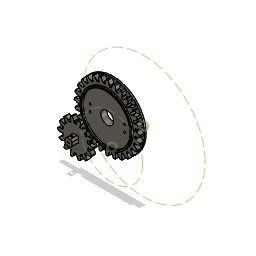
Gears v2 v7 (Autodesk Fusion 360 design; units mm, degrees)
description: Spur Gear; Module: 12.7; Num Teeth: 28; Pressure Angle: 20.0; Backlash: 0.00 mm
description: Spur Gear; Module: 12.7; Num Teeth: 14; Pressure Angle: 20.0; Backlash: 0.00 mm
Autodesk Fusion 360 part; units mm, degrees
(part 1 of 11)
sketch "Sketch1" plane through (0, 0, 0) normal (0, 0, 1) x (1, 0, 0)
  line L0 (-152.4, 152.4) -> (152.4, 152.4)
  line L1 (152.4, 152.4) -> (152.4, -152.4)
  line L2 (152.4, -152.4) -> (-152.4, -152.4)
  line L3 (-152.4, -152.4) -> (-152.4, 152.4)
  line L4 (-152.4, 152.4) -> (152.4, -152.4)
  dimension "d25" = 304.8
  dimension "d26" = 304.8
  constraint horizontal L0
  constraint vertical L1
  constraint horizontal L2
  constraint vertical L3
  constraint midpoint origin L4
  measures "d25" distance of L0.start L0.end
  measures "d26" distance of L0.end L1.end
sketch "Sketch1 (2)" plane through (0, 0, 0) normal (0, 0, 1) x (1, 0, 0) in component "Spur Gear (28 teeth)"
  circle A0 centre (0, 0) radius 162.5092
  circle A1 centre (0, 0) radius 31
extrude "Extrude1" add sketch "Sketch1 (2)" along normal blind 25 makes body 1 in component "Spur Gear (28 teeth)"
sketch "Sketch2" plane through (0, 0, 0) normal (0, 0, 1) x (1, 0, 0) in component "Spur Gear (28 teeth)"
  spline S0 degree 5 poles (166.6564, -11.8532) (166.7254, -11.8581) (166.8636, -11.8663) (167.071, -11.8735) (167.3475, -11.8735) (167.6934, -11.8606) (168.0395, -11.8383) (168.3856, -11.8103) (168.7317, -11.7791) (169.0778, -11.7459) (169.4239, -11.7106) (169.7699, -11.6722) (170.1158, -11.63) (170.4617, -11.5833) (170.8074, -11.5321) (171.153, -11.4767) (171.4984, -11.4177) (171.8437, -11.3558) (172.1889, -11.2914) (172.5338, -11.2245) (172.8787, -11.1552) (173.2233, -11.0833) (173.5677, -11.0087) (173.912, -10.9313) (174.256, -10.8512) (174.5999, -10.7684) (174.9435, -10.6832) (175.2869, -10.5956) (175.6301, -10.5057) (175.973, -10.4136) (176.3158, -10.3193) (176.6582, -10.2229) (177.0005, -10.1242) (177.3424, -10.0233) (177.6842, -9.9203) (178.0256, -9.8151) (178.3669, -9.7079) (178.7078, -9.5986) (179.0485, -9.4873) (179.3888, -9.374) (179.729, -9.2588) (180.0688, -9.1417) (180.4083, -9.0226) (180.7476, -8.9017) (181.0865, -8.7788) (181.4252, -8.6541) (181.7635, -8.5275) (182.1016, -8.3991) (182.4393, -8.269) (182.7767, -8.137) (183.1138, -8.0033) (183.4506, -7.8678) (183.7871, -7.7306) (184.1232, -7.5916) (184.459, -7.451) (184.7945, -7.3086) (185.1296, -7.1646) (185.4644, -7.0189) (185.7989, -6.8716) (186.133, -6.7226) (186.4667, -6.572) (186.8001, -6.4197) (187.1332, -6.2659) (187.4659, -6.1105) (187.7982, -5.9535) (188.1302, -5.7949) (188.4618, -5.6348) (188.793, -5.4731) (189.1239, -5.3099) (189.4544, -5.1452) (189.7845, -4.979) (190.0482, -4.8448) (190.2459, -4.7434) (190.3776, -4.6756) (190.4434, -4.6415) knots 0 0 0 0 0 0 0.01428571 0.02857143 0.04285714 0.05714286 0.07142857 0.08571429 0.1 0.11428571 0.12857143 0.14285714 0.15714286 0.17142857 0.18571429 0.2 0.21428571 0.22857143 0.24285714 0.25714286 0.27142857 0.28571429 0.3 0.31428571 0.32857143 0.34285714 0.35714286 0.37142857 0.38571429 0.4 0.41428571 0.42857143 0.44285714 0.45714286 0.47142857 0.48571429 0.5 0.51428571 0.52857143 0.54285714 0.55714286 0.57142857 0.58571429 0.6 0.61428571 0.62857143 0.64285714 0.65714286 0.67142857 0.68571429 0.7 0.71428571 0.72857143 0.74285714 0.75714286 0.77142857 0.78571429 0.8 0.81428571 0.82857143 0.84285714 0.85714286 0.87142857 0.88571429 0.9 0.91428571 0.92857143 0.94285714 0.95714286 0.97142857 0.98571429 1 1 1 1 1 1
  spline S1 degree 5 poles (166.6564, 11.8532) (166.7254, 11.8581) (166.8636, 11.8663) (167.071, 11.8735) (167.3475, 11.8735) (167.6934, 11.8606) (168.0395, 11.8383) (168.3856, 11.8103) (168.7317, 11.7791) (169.0778, 11.7459) (169.4239, 11.7106) (169.7699, 11.6722) (170.1158, 11.63) (170.4617, 11.5833) (170.8074, 11.5321) (171.153, 11.4767) (171.4984, 11.4177) (171.8437, 11.3558) (172.1889, 11.2914) (172.5338, 11.2245) (172.8787, 11.1552) (173.2233, 11.0833) (173.5677, 11.0087) (173.912, 10.9313) (174.256, 10.8512) (174.5999, 10.7684) (174.9435, 10.6832) (175.2869, 10.5956) (175.6301, 10.5057) (175.973, 10.4136) (176.3158, 10.3193) (176.6582, 10.2229) (177.0005, 10.1242) (177.3424, 10.0233) (177.6842, 9.9203) (178.0256, 9.8151) (178.3669, 9.7079) (178.7078, 9.5986) (179.0485, 9.4873) (179.3888, 9.374) (179.729, 9.2588) (180.0688, 9.1417) (180.4083, 9.0226) (180.7476, 8.9017) (181.0865, 8.7788) (181.4252, 8.6541) (181.7635, 8.5275) (182.1016, 8.3991) (182.4393, 8.269) (182.7767, 8.137) (183.1138, 8.0033) (183.4506, 7.8678) (183.7871, 7.7306) (184.1232, 7.5916) (184.459, 7.451) (184.7945, 7.3086) (185.1296, 7.1646) (185.4644, 7.0189) (185.7989, 6.8716) (186.133, 6.7226) (186.4667, 6.572) (186.8001, 6.4197) (187.1332, 6.2659) (187.4659, 6.1105) (187.7982, 5.9535) (188.1302, 5.7949) (188.4618, 5.6348) (188.793, 5.4731) (189.1239, 5.3099) (189.4544, 5.1452) (189.7845, 4.979) (190.0482, 4.8448) (190.2459, 4.7434) (190.3776, 4.6756) (190.4434, 4.6415) knots 0 0 0 0 0 0 0.01428571 0.02857143 0.04285714 0.05714286 0.07142857 0.08571429 0.1 0.11428571 0.12857143 0.14285714 0.15714286 0.17142857 0.18571429 0.2 0.21428571 0.22857143 0.24285714 0.25714286 0.27142857 0.28571429 0.3 0.31428571 0.32857143 0.34285714 0.35714286 0.37142857 0.38571429 0.4 0.41428571 0.42857143 0.44285714 0.45714286 0.47142857 0.48571429 0.5 0.51428571 0.52857143 0.54285714 0.55714286 0.57142857 0.58571429 0.6 0.61428571 0.62857143 0.64285714 0.65714286 0.67142857 0.68571429 0.7 0.71428571 0.72857143 0.74285714 0.75714286 0.77142857 0.78571429 0.8 0.81428571 0.82857143 0.84285714 0.85714286 0.87142857 0.88571429 0.9 0.91428571 0.92857143 0.94285714 0.95714286 0.97142857 0.98571429 1 1 1 1 1 1
  arc A0 (190.4434, -4.6415) -> (190.4434, 4.6415) centre (0, 0) ccw
  line L0 (162.0897, -11.5292) -> (166.6564, -11.8532)
  line L1 (162.0897, 11.5292) -> (166.6564, 11.8532)
  line L2 (162.0897, -11.5292) -> (162.0897, 11.5292)
  point P0 (168.3364, -11.8136)
  point P1 (170.0254, -11.6404)
  point P2 (171.72, -11.3777)
  point P3 (173.4184, -11.0406)
  point P4 (175.1198, -10.6379)
  point P5 (176.8231, -10.175)
  point P6 (178.5277, -9.656)
  point P7 (180.2329, -9.0839)
  point P8 (181.9381, -8.461)
  point P9 (183.6427, -7.7892)
  point P10 (185.3461, -7.0702)
  point P11 (187.0477, -6.3051)
  point P12 (188.747, -5.4953)
  point P13 (168.3364, 11.8136)
  point P14 (170.0254, 11.6404)
  point P15 (171.72, 11.3777)
  point P16 (173.4184, 11.0406)
  point P17 (175.1198, 10.6379)
  point P18 (176.8231, 10.175)
  point P19 (178.5277, 9.656)
  point P20 (180.2329, 9.0839)
  point P21 (181.9381, 8.461)
  point P22 (183.6427, 7.7892)
  point P23 (185.3461, 7.0702)
  point P24 (187.0477, 6.3051)
  point P25 (188.747, 5.4953)
extrude "Extrude2" add sketch "Sketch2" along normal blind 25 bodies 1 in component "Spur Gear (28 teeth)"
fillet "Fillet1" radius 1.5875 2 edges at (162.0997, -11.5299, 12.5) (162.0997, 11.5299, 12.5) on bodies 1 in component "Spur Gear (28 teeth)"
pattern_circular "C-Pattern1" count 28 over 360 about axis through (0, 0, 0) along (0, 0, 1) of "Extrude2", "Fillet1" in component "Spur Gear (28 teeth)"
sketch "Sketch3" plane through (0, 0, 0) normal (0, 0, 1) x (1, 0, 0) in component "Spur Gear (28 teeth)"
  circle A0 centre (0, 0) radius 177.8 construction
sketch "Sketch1 (3)" plane through (0, 0, 0) normal (0, 0, 1) x (1, 0, 0) in component "Spur Gear (14 teeth)"
  circle A0 centre (0, 0) radius 73.6092
  circle A1 centre (0, 0) radius 10
extrude "Extrude1'" add sketch "Sketch1 (3)" along normal blind 25 separate body makes body 2 in component "Spur Gear (14 teeth)"
sketch "Sketch2 (2)" plane through (0, 0, 0) normal (0, 0, 1) x (1, 0, 0) in component "Spur Gear (14 teeth)"
  spline S0 degree 5 poles (82.8648, -10.5895) (82.9186, -10.5964) (83.0264, -10.6085) (83.1884, -10.6217) (83.4049, -10.6299) (83.6763, -10.6275) (83.9482, -10.6159) (84.2204, -10.5989) (84.4927, -10.5788) (84.7651, -10.5568) (85.0375, -10.5325) (85.31, -10.5051) (85.5825, -10.4738) (85.855, -10.438) (86.1276, -10.3977) (86.4002, -10.3533) (86.6727, -10.3055) (86.9452, -10.2547) (87.2175, -10.2014) (87.4897, -10.1457) (87.7618, -10.0875) (88.0338, -10.0267) (88.3056, -9.9631) (88.5772, -9.8967) (88.8487, -9.8275) (89.12, -9.7558) (89.3911, -9.6815) (89.6621, -9.6048) (89.9328, -9.5259) (90.2032, -9.4447) (90.4735, -9.3613) (90.7435, -9.2757) (91.0132, -9.1878) (91.2827, -9.0976) (91.5519, -9.0053) (91.8209, -8.9108) (92.0895, -8.8142) (92.3579, -8.7155) (92.626, -8.6148) (92.8938, -8.5121) (93.1612, -8.4074) (93.4284, -8.3007) (93.6952, -8.192) (93.9617, -8.0814) (94.2278, -7.9688) (94.4936, -7.8544) (94.7591, -7.738) (95.0241, -7.6198) (95.2889, -7.4998) (95.5532, -7.3779) (95.8172, -7.2542) (96.0808, -7.1287) (96.3439, -7.0014) (96.6067, -6.8723) (96.8691, -6.7415) (97.1311, -6.6089) (97.3927, -6.4747) (97.6539, -6.3387) (97.9146, -6.201) (98.1749, -6.0616) (98.4348, -5.9205) (98.6942, -5.7778) (98.9532, -5.6334) (99.2117, -5.4874) (99.4698, -5.3397) (99.7274, -5.1905) (99.9845, -5.0396) (100.2412, -4.8871) (100.4974, -4.7331) (100.7531, -4.5775) (101.0083, -4.4203) (101.2121, -4.2933) (101.3647, -4.1974) (101.4664, -4.1331) (101.5172, -4.1009) knots 0 0 0 0 0 0 0.01428571 0.02857143 0.04285714 0.05714286 0.07142857 0.08571429 0.1 0.11428571 0.12857143 0.14285714 0.15714286 0.17142857 0.18571429 0.2 0.21428571 0.22857143 0.24285714 0.25714286 0.27142857 0.28571429 0.3 0.31428571 0.32857143 0.34285714 0.35714286 0.37142857 0.38571429 0.4 0.41428571 0.42857143 0.44285714 0.45714286 0.47142857 0.48571429 0.5 0.51428571 0.52857143 0.54285714 0.55714286 0.57142857 0.58571429 0.6 0.61428571 0.62857143 0.64285714 0.65714286 0.67142857 0.68571429 0.7 0.71428571 0.72857143 0.74285714 0.75714286 0.77142857 0.78571429 0.8 0.81428571 0.82857143 0.84285714 0.85714286 0.87142857 0.88571429 0.9 0.91428571 0.92857143 0.94285714 0.95714286 0.97142857 0.98571429 1 1 1 1 1 1
  spline S1 degree 5 poles (82.8648, 10.5895) (82.9186, 10.5964) (83.0264, 10.6085) (83.1884, 10.6217) (83.4049, 10.6299) (83.6763, 10.6275) (83.9482, 10.6159) (84.2204, 10.5989) (84.4927, 10.5788) (84.7651, 10.5568) (85.0375, 10.5325) (85.31, 10.5051) (85.5825, 10.4738) (85.855, 10.438) (86.1276, 10.3977) (86.4002, 10.3533) (86.6727, 10.3055) (86.9452, 10.2547) (87.2175, 10.2014) (87.4897, 10.1457) (87.7618, 10.0875) (88.0338, 10.0267) (88.3056, 9.9631) (88.5772, 9.8967) (88.8487, 9.8275) (89.12, 9.7558) (89.3911, 9.6815) (89.6621, 9.6048) (89.9328, 9.5259) (90.2032, 9.4447) (90.4735, 9.3613) (90.7435, 9.2757) (91.0132, 9.1878) (91.2827, 9.0976) (91.5519, 9.0053) (91.8209, 8.9108) (92.0895, 8.8142) (92.3579, 8.7155) (92.626, 8.6148) (92.8938, 8.5121) (93.1612, 8.4074) (93.4284, 8.3007) (93.6952, 8.192) (93.9617, 8.0814) (94.2278, 7.9688) (94.4936, 7.8544) (94.7591, 7.738) (95.0241, 7.6198) (95.2889, 7.4998) (95.5532, 7.3779) (95.8172, 7.2542) (96.0808, 7.1287) (96.3439, 7.0014) (96.6067, 6.8723) (96.8691, 6.7415) (97.1311, 6.6089) (97.3927, 6.4747) (97.6539, 6.3387) (97.9146, 6.201) (98.1749, 6.0616) (98.4348, 5.9205) (98.6942, 5.7778) (98.9532, 5.6334) (99.2117, 5.4874) (99.4698, 5.3397) (99.7274, 5.1905) (99.9845, 5.0396) (100.2412, 4.8871) (100.4974, 4.7331) (100.7531, 4.5775) (101.0083, 4.4203) (101.2121, 4.2933) (101.3647, 4.1974) (101.4664, 4.1331) (101.5172, 4.1009) knots 0 0 0 0 0 0 0.01428571 0.02857143 0.04285714 0.05714286 0.07142857 0.08571429 0.1 0.11428571 0.12857143 0.14285714 0.15714286 0.17142857 0.18571429 0.2 0.21428571 0.22857143 0.24285714 0.25714286 0.27142857 0.28571429 0.3 0.31428571 0.32857143 0.34285714 0.35714286 0.37142857 0.38571429 0.4 0.41428571 0.42857143 0.44285714 0.45714286 0.47142857 0.48571429 0.5 0.51428571 0.52857143 0.54285714 0.55714286 0.57142857 0.58571429 0.6 0.61428571 0.62857143 0.64285714 0.65714286 0.67142857 0.68571429 0.7 0.71428571 0.72857143 0.74285714 0.75714286 0.77142857 0.78571429 0.8 0.81428571 0.82857143 0.84285714 0.85714286 0.87142857 0.88571429 0.9 0.91428571 0.92857143 0.94285714 0.95714286 0.97142857 0.98571429 1 1 1 1 1 1
  arc A0 (101.5172, -4.1009) -> (101.5172, 4.1009) centre (0, 0) ccw
  line L0 (73.0055, -9.3309) -> (82.8648, -10.5895)
  line L1 (73.0055, 9.3309) -> (82.8648, 10.5895)
  line L2 (73.0055, -9.3309) -> (73.0055, 9.3309)
  point P0 (84.1637, -10.6019)
  point P1 (85.4782, -10.4853)
  point P2 (86.8022, -10.281)
  point P3 (88.1332, -10.003)
  point P4 (89.4693, -9.659)
  point P5 (90.8089, -9.254)
  point P6 (92.1509, -8.7913)
  point P7 (93.4941, -8.2736)
  point P8 (94.8372, -7.7029)
  point P9 (96.1793, -7.0807)
  point P10 (97.5194, -6.4084)
  point P11 (98.8564, -5.6871)
  point P12 (100.1893, -4.9177)
  point P13 (84.1637, 10.6019)
  point P14 (85.4782, 10.4853)
  point P15 (86.8022, 10.281)
  point P16 (88.1332, 10.003)
  point P17 (89.4693, 9.659)
  point P18 (90.8089, 9.254)
  point P19 (92.1509, 8.7913)
  point P20 (93.4941, 8.2736)
  point P21 (94.8372, 7.7029)
  point P22 (96.1793, 7.0807)
  point P23 (97.5194, 6.4084)
  point P24 (98.8564, 5.6871)
  point P25 (100.1893, 4.9177)
extrude "Extrude2'" add sketch "Sketch2 (2)" along normal blind 25 bodies 2 in component "Spur Gear (14 teeth)"
fillet "Fillet1'" radius 1.5875 2 edges at (73.0152, -9.3321, 12.5) (73.0152, 9.3321, 12.5) on bodies 2 in component "Spur Gear (14 teeth)"
pattern_circular "C-Pattern1'" count 14 over 360 about axis through (0, 0, 0) along (0, 0, 1) of "Extrude2'", "Fillet1'" in component "Spur Gear (14 teeth)"
sketch "Sketch3 (2)" plane through (0, 0, 0) normal (0, 0, 1) x (1, 0, 0) in component "Spur Gear (14 teeth)"
  circle A0 centre (0, 0) radius 88.9 construction
scale "Scale1" factor 0.5 about (-161.9806, -13.0972, 25) bodies 1 in component "Spur Gear (28 teeth)"
scale "Scale1'" factor 0.5 about (-161.9806, -13.0972, 25) bodies 2 in component "Spur Gear (14 teeth)"
sketch "Sketch2 (3)" plane through (0, 0, 25) normal (0, 0, 1) x (1, 0, 0)
  arc A0 (79.8631, -10.983) -> (80.4364, -5.894) centre (-0.5538, 0.6546) ccw
  arc A1 (81.2838, -5.1662) -> (80.4364, -5.894) centre (81.2276, -5.958) ccw
  line L0 (81.2838, -5.1662) -> (82.7743, -5.272)
  spline S0 degree 5 poles (82.7743, -5.272) (82.8089, -5.2744) (82.878, -5.2785) (82.9816, -5.2821) (83.1199, -5.2821) (83.2929, -5.2756) (83.4659, -5.2645) (83.6389, -5.2505) (83.812, -5.2349) (83.9851, -5.2183) (84.1581, -5.2006) (84.3311, -5.1815) (84.5041, -5.1604) (84.677, -5.137) (84.8498, -5.1114) (85.0226, -5.0837) (85.1954, -5.0542) (85.368, -5.0233) (85.5406, -4.991) (85.7131, -4.9576) (85.8855, -4.9229) (86.0578, -4.887) (86.23, -4.8497) (86.4021, -4.811) (86.5742, -4.7709) (86.7461, -4.7296) (86.9179, -4.6869) (87.0896, -4.6431) (87.2612, -4.5982) (87.4327, -4.5522) (87.604, -4.505) (87.7753, -4.4568) (87.9464, -4.4075) (88.1174, -4.357) (88.2882, -4.3055) (88.459, -4.2529) (88.6296, -4.1993) (88.8001, -4.1446) (88.9704, -4.089) (89.1406, -4.0324) (89.3106, -3.9748) (89.4806, -3.9162) (89.6503, -3.8567) (89.8199, -3.7962) (89.9894, -3.7348) (90.1588, -3.6724) (90.3279, -3.6091) (90.4969, -3.5449) (90.6658, -3.4798) (90.8345, -3.4139) (91.0031, -3.347) (91.1715, -3.2793) (91.3397, -3.2106) (91.5078, -3.1412) (91.6757, -3.0708) (91.8434, -2.9997) (92.011, -2.9277) (92.1784, -2.8548) (92.3456, -2.7811) (92.5127, -2.7067) (92.6795, -2.6313) (92.8462, -2.5552) (93.0128, -2.4783) (93.1791, -2.4006) (93.3453, -2.3221) (93.5113, -2.2428) (93.6771, -2.1628) (93.8427, -2.0819) (94.0081, -2.0003) (94.1733, -1.918) (94.3384, -1.8348) (94.4703, -1.7677) (94.5691, -1.7171) (94.635, -1.6831) (94.6679, -1.6661) knots 0 0 0 0 0 0 0.01428571 0.02857143 0.04285714 0.05714286 0.07142857 0.08571429 0.1 0.11428571 0.12857143 0.14285714 0.15714286 0.17142857 0.18571429 0.2 0.21428571 0.22857143 0.24285714 0.25714286 0.27142857 0.28571429 0.3 0.31428571 0.32857143 0.34285714 0.35714286 0.37142857 0.38571429 0.4 0.41428571 0.42857143 0.44285714 0.45714286 0.47142857 0.48571429 0.5 0.51428571 0.52857143 0.54285714 0.55714286 0.57142857 0.58571429 0.6 0.61428571 0.62857143 0.64285714 0.65714286 0.67142857 0.68571429 0.7 0.71428571 0.72857143 0.74285714 0.75714286 0.77142857 0.78571429 0.8 0.81428571 0.82857143 0.84285714 0.85714286 0.87142857 0.88571429 0.9 0.91428571 0.92857143 0.94285714 0.95714286 0.97142857 0.98571429 1 1 1 1 1 1
  arc A2 (94.6679, -1.6661) -> (94.6679, 2.9754) centre (-0.5538, 0.6546) ccw
  spline S1 degree 5 poles (94.6679, 2.9754) (94.635, 2.9924) (94.5691, 3.0263) (94.4703, 3.077) (94.3384, 3.1441) (94.1733, 3.2272) (94.0081, 3.3096) (93.8427, 3.3912) (93.6771, 3.472) (93.5113, 3.5521) (93.3453, 3.6314) (93.1791, 3.7099) (93.0128, 3.7876) (92.8462, 3.8645) (92.6795, 3.9406) (92.5127, 4.0159) (92.3456, 4.0904) (92.1784, 4.1641) (92.011, 4.2369) (91.8434, 4.3089) (91.6757, 4.3801) (91.5078, 4.4504) (91.3397, 4.5199) (91.1715, 4.5885) (91.0031, 4.6563) (90.8345, 4.7231) (90.6658, 4.7891) (90.4969, 4.8542) (90.3279, 4.9184) (90.1588, 4.9817) (89.9894, 5.044) (89.8199, 5.1055) (89.6503, 5.166) (89.4806, 5.2255) (89.3106, 5.2841) (89.1406, 5.3417) (88.9704, 5.3983) (88.8001, 5.4539) (88.6296, 5.5086) (88.459, 5.5622) (88.2882, 5.6148) (88.1174, 5.6663) (87.9464, 5.7167) (87.7753, 5.7661) (87.604, 5.8143) (87.4327, 5.8615) (87.2612, 5.9075) (87.0896, 5.9524) (86.9179, 5.9962) (86.7461, 6.0388) (86.5742, 6.0802) (86.4021, 6.1203) (86.23, 6.159) (86.0578, 6.1963) (85.8855, 6.2322) (85.7131, 6.2669) (85.5406, 6.3003) (85.368, 6.3326) (85.1954, 6.3635) (85.0226, 6.393) (84.8498, 6.4207) (84.677, 6.4463) (84.5041, 6.4697) (84.3311, 6.4908) (84.1581, 6.5099) (83.9851, 6.5276) (83.812, 6.5442) (83.6389, 6.5598) (83.4659, 6.5738) (83.2929, 6.5849) (83.1199, 6.5914) (82.9816, 6.5914) (82.878, 6.5878) (82.8089, 6.5837) (82.7743, 6.5813) knots -1 -1 -1 -1 -1 -1 -0.98571429 -0.97142857 -0.95714286 -0.94285714 -0.92857143 -0.91428571 -0.9 -0.88571429 -0.87142857 -0.85714286 -0.84285714 -0.82857143 -0.81428571 -0.8 -0.78571429 -0.77142857 -0.75714286 -0.74285714 -0.72857143 -0.71428571 -0.7 -0.68571429 -0.67142857 -0.65714286 -0.64285714 -0.62857143 -0.61428571 -0.6 -0.58571429 -0.57142857 -0.55714286 -0.54285714 -0.52857143 -0.51428571 -0.5 -0.48571429 -0.47142857 -0.45714286 -0.44285714 -0.42857143 -0.41428571 -0.4 -0.38571429 -0.37142857 -0.35714286 -0.34285714 -0.32857143 -0.31428571 -0.3 -0.28571429 -0.27142857 -0.25714286 -0.24285714 -0.22857143 -0.21428571 -0.2 -0.18571429 -0.17142857 -0.15714286 -0.14285714 -0.12857143 -0.11428571 -0.1 -0.08571429 -0.07142857 -0.05714286 -0.04285714 -0.02857143 -0.01428571 0 0 0 0 0 0
  line L1 (82.7743, 6.5813) -> (81.2838, 6.4755)
  arc A3 (80.4364, 7.2033) -> (81.2838, 6.4755) centre (81.2276, 7.2672) ccw
  arc A4 (80.4364, 7.2033) -> (79.8631, 12.2922) centre (-0.5538, 0.6546) ccw
  arc A5 (80.5272, 13.1903) -> (79.8631, 12.2922) centre (80.6486, 12.4059) ccw
  line L2 (80.5272, 13.1903) -> (82.0039, 13.4189)
  spline S2 degree 5 poles (82.0039, 13.4189) (82.0381, 13.4242) (82.1064, 13.4356) (82.2083, 13.4551) (82.3431, 13.4859) (82.5103, 13.5307) (82.6765, 13.5801) (82.8421, 13.6322) (83.0073, 13.6859) (83.1724, 13.7406) (83.3371, 13.7963) (83.5015, 13.8535) (83.6655, 13.9126) (83.8288, 13.9738) (83.9917, 14.0373) (84.154, 14.1027) (84.3158, 14.1699) (84.4772, 14.2385) (84.6383, 14.3083) (84.799, 14.3793) (84.9594, 14.4515) (85.1194, 14.5248) (85.279, 14.5995) (85.4382, 14.6756) (85.597, 14.7529) (85.7554, 14.8315) (85.9134, 14.9113) (86.0711, 14.9922) (86.2284, 15.0742) (86.3853, 15.1572) (86.5419, 15.2413) (86.6981, 15.3264) (86.8539, 15.4126) (87.0094, 15.4998) (87.1645, 15.5881) (87.3193, 15.6774) (87.4737, 15.7676) (87.6277, 15.8588) (87.7814, 15.9509) (87.9347, 16.044) (88.0877, 16.138) (88.2403, 16.2329) (88.3926, 16.3287) (88.5445, 16.4255) (88.6961, 16.5231) (88.8473, 16.6215) (88.9981, 16.7209) (89.1486, 16.8211) (89.2988, 16.9221) (89.4486, 17.024) (89.598, 17.1267) (89.7471, 17.2302) (89.8958, 17.3345) (90.0442, 17.4396) (90.1923, 17.5456) (90.34, 17.6523) (90.4873, 17.7598) (90.6343, 17.868) (90.7809, 17.9771) (90.9272, 18.0869) (91.0732, 18.1974) (91.2188, 18.3087) (91.364, 18.4208) (91.5089, 18.5335) (91.6534, 18.647) (91.7976, 18.7613) (91.9414, 18.8762) (92.0849, 18.9919) (92.228, 19.1082) (92.3708, 19.2253) (92.5132, 19.3431) (92.6269, 19.4379) (92.7119, 19.5092) (92.7686, 19.557) (92.7969, 19.5809) knots 0 0 0 0 0 0 0.01428571 0.02857143 0.04285714 0.05714286 0.07142857 0.08571429 0.1 0.11428571 0.12857143 0.14285714 0.15714286 0.17142857 0.18571429 0.2 0.21428571 0.22857143 0.24285714 0.25714286 0.27142857 0.28571429 0.3 0.31428571 0.32857143 0.34285714 0.35714286 0.37142857 0.38571429 0.4 0.41428571 0.42857143 0.44285714 0.45714286 0.47142857 0.48571429 0.5 0.51428571 0.52857143 0.54285714 0.55714286 0.57142857 0.58571429 0.6 0.61428571 0.62857143 0.64285714 0.65714286 0.67142857 0.68571429 0.7 0.71428571 0.72857143 0.74285714 0.75714286 0.77142857 0.78571429 0.8 0.81428571 0.82857143 0.84285714 0.85714286 0.87142857 0.88571429 0.9 0.91428571 0.92857143 0.94285714 0.95714286 0.97142857 0.98571429 1 1 1 1 1 1
  arc A6 (92.7969, 19.5809) -> (91.7641, 24.1061) centre (-0.5538, 0.6546) ccw
  spline S3 degree 5 poles (91.7641, 24.1061) (91.7282, 24.1153) (91.6564, 24.1337) (91.5488, 24.1611) (91.4053, 24.1972) (91.2259, 24.2415) (91.0464, 24.2851) (90.867, 24.3278) (90.6876, 24.3697) (90.5081, 24.4109) (90.3286, 24.4513) (90.1492, 24.4908) (89.9697, 24.5296) (89.7902, 24.5675) (89.6108, 24.6046) (89.4313, 24.6409) (89.2519, 24.6763) (89.0725, 24.711) (88.893, 24.7447) (88.7137, 24.7777) (88.5343, 24.8097) (88.3549, 24.8409) (88.1756, 24.8712) (87.9964, 24.9007) (87.8171, 24.9293) (87.6379, 24.957) (87.4587, 24.9837) (87.2796, 25.0096) (87.1006, 25.0346) (86.9215, 25.0586) (86.7426, 25.0818) (86.5637, 25.1039) (86.3849, 25.1252) (86.2061, 25.1454) (86.0274, 25.1647) (85.8488, 25.183) (85.6703, 25.2004) (85.4918, 25.2167) (85.3135, 25.232) (85.1352, 25.2464) (84.9571, 25.2596) (84.779, 25.2718) (84.6011, 25.283) (84.4233, 25.293) (84.2456, 25.3019) (84.068, 25.3097) (83.8906, 25.3165) (83.7133, 25.3221) (83.5362, 25.3266) (83.3592, 25.3299) (83.1824, 25.332) (83.0058, 25.3328) (82.8293, 25.3322) (82.6531, 25.3302) (82.4771, 25.3269) (82.3013, 25.3224) (82.1257, 25.3166) (81.9503, 25.3096) (81.7751, 25.3014) (81.6002, 25.2917) (81.4255, 25.2802) (81.2513, 25.2667) (81.0775, 25.251) (80.9042, 25.2331) (80.7313, 25.2133) (80.5586, 25.192) (80.3862, 25.1697) (80.214, 25.1464) (80.0422, 25.1215) (79.8711, 25.0939) (79.701, 25.0617) (79.5662, 25.0309) (79.4659, 25.0043) (79.3995, 24.985) (79.3663, 24.9749) knots -1 -1 -1 -1 -1 -1 -0.98571429 -0.97142857 -0.95714286 -0.94285714 -0.92857143 -0.91428571 -0.9 -0.88571429 -0.87142857 -0.85714286 -0.84285714 -0.82857143 -0.81428571 -0.8 -0.78571429 -0.77142857 -0.75714286 -0.74285714 -0.72857143 -0.71428571 -0.7 -0.68571429 -0.67142857 -0.65714286 -0.64285714 -0.62857143 -0.61428571 -0.6 -0.58571429 -0.57142857 -0.55714286 -0.54285714 -0.52857143 -0.51428571 -0.5 -0.48571429 -0.47142857 -0.45714286 -0.44285714 -0.42857143 -0.41428571 -0.4 -0.38571429 -0.37142857 -0.35714286 -0.34285714 -0.32857143 -0.31428571 -0.3 -0.28571429 -0.27142857 -0.25714286 -0.24285714 -0.22857143 -0.21428571 -0.2 -0.18571429 -0.17142857 -0.15714286 -0.14285714 -0.12857143 -0.11428571 -0.1 -0.08571429 -0.07142857 -0.05714286 -0.04285714 -0.02857143 -0.01428571 0 0 0 0 0 0
  line L3 (79.3663, 24.9749) -> (77.9367, 24.5401)
  arc A7 (76.9486, 25.0611) -> (77.9367, 24.5401) centre (77.7057, 25.2995) ccw
  arc A8 (76.9486, 25.0611) -> (75.2572, 29.8949) centre (-0.5538, 0.6546) ccw
  arc A9 (75.7049, 30.9183) -> (75.2572, 29.8949) centre (75.9978, 30.1805) ccw
  line L4 (75.7049, 30.9183) -> (77.0937, 31.4697)
  spline S4 degree 5 poles (77.0937, 31.4697) (77.1259, 31.4825) (77.1899, 31.5088) (77.2849, 31.5505) (77.4095, 31.6105) (77.5625, 31.6914) (77.7135, 31.7765) (77.8634, 31.8642) (78.0125, 31.9533) (78.1613, 32.0433) (78.3095, 32.1344) (78.4571, 32.2267) (78.6037, 32.3207) (78.7494, 32.4168) (78.894, 32.5149) (79.0377, 32.6148) (79.1805, 32.7163) (79.3226, 32.8191) (79.4641, 32.923) (79.605, 33.028) (79.7453, 33.134) (79.885, 33.2412) (80.024, 33.3495) (80.1623, 33.4591) (80.2999, 33.5698) (80.4368, 33.6817) (80.5731, 33.7946) (80.7088, 33.9086) (80.8439, 34.0235) (80.9784, 34.1394) (81.1124, 34.2562) (81.2457, 34.374) (81.3785, 34.4927) (81.5106, 34.6123) (81.6422, 34.7329) (81.7732, 34.8543) (81.9037, 34.9766) (82.0336, 35.0998) (82.1629, 35.2239) (82.2917, 35.3487) (82.4199, 35.4744) (82.5476, 35.6009) (82.6747, 35.7282) (82.8013, 35.8563) (82.9273, 35.9852) (83.0528, 36.1148) (83.1778, 36.2452) (83.3022, 36.3764) (83.4261, 36.5083) (83.5495, 36.641) (83.6723, 36.7743) (83.7947, 36.9084) (83.9165, 37.0433) (84.0377, 37.1788) (84.1585, 37.315) (84.2787, 37.4519) (84.3985, 37.5895) (84.5177, 37.7277) (84.6364, 37.8667) (84.7546, 38.0063) (84.8723, 38.1465) (84.9894, 38.2874) (85.1061, 38.429) (85.2222, 38.5712) (85.3379, 38.714) (85.453, 38.8574) (85.5677, 39.0015) (85.6818, 39.1462) (85.7955, 39.2915) (85.9086, 39.4374) (86.0212, 39.5839) (86.111, 39.7016) (86.178, 39.7901) (86.2226, 39.8493) (86.2449, 39.8789) knots 0 0 0 0 0 0 0.01428571 0.02857143 0.04285714 0.05714286 0.07142857 0.08571429 0.1 0.11428571 0.12857143 0.14285714 0.15714286 0.17142857 0.18571429 0.2 0.21428571 0.22857143 0.24285714 0.25714286 0.27142857 0.28571429 0.3 0.31428571 0.32857143 0.34285714 0.35714286 0.37142857 0.38571429 0.4 0.41428571 0.42857143 0.44285714 0.45714286 0.47142857 0.48571429 0.5 0.51428571 0.52857143 0.54285714 0.55714286 0.57142857 0.58571429 0.6 0.61428571 0.62857143 0.64285714 0.65714286 0.67142857 0.68571429 0.7 0.71428571 0.72857143 0.74285714 0.75714286 0.77142857 0.78571429 0.8 0.81428571 0.82857143 0.84285714 0.85714286 0.87142857 0.88571429 0.9 0.91428571 0.92857143 0.94285714 0.95714286 0.97142857 0.98571429 1 1 1 1 1 1
  arc A10 (86.2449, 39.8789) -> (84.231, 44.0607) centre (-0.5538, 0.6546) ccw
  spline S5 degree 5 poles (84.231, 44.0607) (84.194, 44.0618) (84.1199, 44.0638) (84.0089, 44.0665) (83.861, 44.0698) (83.6762, 44.0731) (83.4916, 44.0756) (83.3071, 44.0773) (83.1228, 44.0783) (82.9387, 44.0785) (82.7548, 44.0779) (82.571, 44.0765) (82.3874, 44.0744) (82.204, 44.0714) (82.0208, 44.0677) (81.8378, 44.0631) (81.6549, 44.0577) (81.4723, 44.0515) (81.2899, 44.0445) (81.1077, 44.0367) (80.9257, 44.0281) (80.7439, 44.0186) (80.5623, 44.0083) (80.381, 43.9971) (80.1998, 43.985) (80.019, 43.9722) (79.8383, 43.9584) (79.658, 43.9438) (79.4778, 43.9283) (79.2979, 43.9119) (79.1183, 43.8946) (78.939, 43.8764) (78.7599, 43.8573) (78.5811, 43.8373) (78.4026, 43.8163) (78.2244, 43.7945) (78.0465, 43.7716) (77.8689, 43.7478) (77.6916, 43.7231) (77.5146, 43.6974) (77.338, 43.6707) (77.1617, 43.643) (76.9858, 43.6142) (76.8102, 43.5844) (76.635, 43.5536) (76.4601, 43.5217) (76.2856, 43.4888) (76.1116, 43.4548) (75.9378, 43.4198) (75.7646, 43.3837) (75.5917, 43.3463) (75.4193, 43.3078) (75.2475, 43.268) (75.0761, 43.2269) (74.9053, 43.1845) (74.7349, 43.1409) (74.565, 43.0962) (74.3955, 43.0504) (74.2265, 43.0033) (74.0581, 42.955) (73.8904, 42.9049) (73.7236, 42.853) (73.5577, 42.799) (73.3927, 42.743) (73.2285, 42.6852) (73.0649, 42.6261) (72.9018, 42.5659) (72.7391, 42.5049) (72.5771, 42.4424) (72.4164, 42.3774) (72.2578, 42.3082) (72.1332, 42.2481) (72.0413, 42.1999) (71.9808, 42.1663) (71.9508, 42.1491) knots -1 -1 -1 -1 -1 -1 -0.98571429 -0.97142857 -0.95714286 -0.94285714 -0.92857143 -0.91428571 -0.9 -0.88571429 -0.87142857 -0.85714286 -0.84285714 -0.82857143 -0.81428571 -0.8 -0.78571429 -0.77142857 -0.75714286 -0.74285714 -0.72857143 -0.71428571 -0.7 -0.68571429 -0.67142857 -0.65714286 -0.64285714 -0.62857143 -0.61428571 -0.6 -0.58571429 -0.57142857 -0.55714286 -0.54285714 -0.52857143 -0.51428571 -0.5 -0.48571429 -0.47142857 -0.45714286 -0.44285714 -0.42857143 -0.41428571 -0.4 -0.38571429 -0.37142857 -0.35714286 -0.34285714 -0.32857143 -0.31428571 -0.3 -0.28571429 -0.27142857 -0.25714286 -0.24285714 -0.22857143 -0.21428571 -0.2 -0.18571429 -0.17142857 -0.15714286 -0.14285714 -0.12857143 -0.11428571 -0.1 -0.08571429 -0.07142857 -0.05714286 -0.04285714 -0.02857143 -0.01428571 0 0 0 0 0 0
  line L5 (71.9508, 42.1491) -> (70.6538, 41.4071)
  arc A11 (69.5745, 41.6951) -> (70.6538, 41.4071) centre (70.2596, 42.096) ccw
  arc A12 (69.5745, 41.6951) -> (66.8499, 46.0313) centre (-0.5538, 0.6546) ccw
  arc A13 (67.0586, 47.1287) -> (66.8499, 46.0313) centre (67.5084, 46.4746) ccw
  line L6 (67.0586, 47.1287) -> (68.2899, 47.9753)
  spline S6 degree 5 poles (68.2899, 47.9753) (68.3185, 47.9949) (68.375, 48.0348) (68.4583, 48.0966) (68.5664, 48.1828) (68.6976, 48.2957) (68.826, 48.4123) (68.9525, 48.5312) (69.0781, 48.6512) (69.2031, 48.7721) (69.3273, 48.8938) (69.4506, 49.0167) (69.5727, 49.141) (69.6933, 49.2671) (69.8125, 49.3949) (69.9303, 49.5243) (70.047, 49.655) (70.1627, 49.7869) (70.2775, 49.9197) (70.3915, 50.0534) (70.5047, 50.1879) (70.617, 50.3235) (70.7284, 50.46) (70.8389, 50.5976) (70.9484, 50.7362) (71.057, 50.8757) (71.1647, 51.0162) (71.2717, 51.1575) (71.3778, 51.2996) (71.4832, 51.4425) (71.5878, 51.5862) (71.6916, 51.7307) (71.7946, 51.8759) (71.8968, 52.022) (71.9983, 52.1688) (72.099, 52.3164) (72.1989, 52.4646) (72.2982, 52.6136) (72.3966, 52.7633) (72.4944, 52.9137) (72.5914, 53.0648) (72.6878, 53.2165) (72.7834, 53.3689) (72.8783, 53.522) (72.9725, 53.6757) (73.066, 53.83) (73.1588, 53.9849) (73.2509, 54.1405) (73.3424, 54.2967) (73.4331, 54.4535) (73.5232, 54.6108) (73.6126, 54.7688) (73.7014, 54.9273) (73.7895, 55.0864) (73.8769, 55.2461) (73.9637, 55.4063) (74.0498, 55.5671) (74.1352, 55.7284) (74.22, 55.8903) (74.3042, 56.0527) (74.3877, 56.2156) (74.4706, 56.3791) (74.5528, 56.543) (74.6344, 56.7075) (74.7154, 56.8725) (74.7958, 57.0379) (74.8755, 57.2039) (74.9545, 57.3704) (75.033, 57.5373) (75.1108, 57.7047) (75.1881, 57.8726) (75.2493, 58.0073) (75.295, 58.1086) (75.3253, 58.1761) (75.3405, 58.21) knots 0 0 0 0 0 0 0.01428571 0.02857143 0.04285714 0.05714286 0.07142857 0.08571429 0.1 0.11428571 0.12857143 0.14285714 0.15714286 0.17142857 0.18571429 0.2 0.21428571 0.22857143 0.24285714 0.25714286 0.27142857 0.28571429 0.3 0.31428571 0.32857143 0.34285714 0.35714286 0.37142857 0.38571429 0.4 0.41428571 0.42857143 0.44285714 0.45714286 0.47142857 0.48571429 0.5 0.51428571 0.52857143 0.54285714 0.55714286 0.57142857 0.58571429 0.6 0.61428571 0.62857143 0.64285714 0.65714286 0.67142857 0.68571429 0.7 0.71428571 0.72857143 0.74285714 0.75714286 0.77142857 0.78571429 0.8 0.81428571 0.82857143 0.84285714 0.85714286 0.87142857 0.88571429 0.9 0.91428571 0.92857143 0.94285714 0.95714286 0.97142857 0.98571429 1 1 1 1 1 1
  arc A14 (75.3405, 58.21) -> (72.4465, 61.8389) centre (-0.5538, 0.6546) ccw
  spline S7 degree 5 poles (72.4465, 61.8389) (72.4102, 61.8316) (72.3375, 61.8171) (72.2287, 61.7951) (72.0837, 61.7653) (71.9029, 61.7274) (71.7223, 61.6888) (71.5421, 61.6494) (71.3622, 61.6094) (71.1827, 61.5686) (71.0035, 61.5271) (70.8246, 61.4849) (70.6461, 61.4419) (70.468, 61.3982) (70.2902, 61.3538) (70.1127, 61.3086) (69.9357, 61.2627) (69.759, 61.216) (69.5827, 61.1686) (69.4068, 61.1204) (69.2313, 61.0715) (69.0562, 61.0218) (68.8815, 60.9713) (68.7072, 60.9201) (68.5333, 60.8681) (68.3598, 60.8152) (68.1868, 60.7616) (68.0141, 60.7072) (67.842, 60.652) (67.6703, 60.596) (67.499, 60.5392) (67.3282, 60.4816) (67.1579, 60.4231) (66.988, 60.3638) (66.8186, 60.3037) (66.6498, 60.2427) (66.4814, 60.1808) (66.3135, 60.1181) (66.1462, 60.0545) (65.9794, 59.9901) (65.8131, 59.9248) (65.6474, 59.8585) (65.4823, 59.7913) (65.3177, 59.7232) (65.1538, 59.6542) (64.9904, 59.5842) (64.8276, 59.5133) (64.6655, 59.4414) (64.5039, 59.3686) (64.343, 59.2948) (64.1828, 59.22) (64.0233, 59.144) (63.8646, 59.067) (63.7067, 58.9887) (63.5496, 58.9094) (63.3932, 58.829) (63.2375, 58.7476) (63.0824, 58.6652) (62.9282, 58.5818) (62.7747, 58.4971) (62.6224, 58.411) (62.4713, 58.3233) (62.3215, 58.2337) (62.1731, 58.1424) (62.0259, 58.0495) (61.8796, 57.9555) (61.7339, 57.8605) (61.5889, 57.7648) (61.4449, 57.6679) (61.3027, 57.5687) (61.1634, 57.4659) (61.0553, 57.3797) (60.9765, 57.3122) (60.925, 57.266) (60.8996, 57.2425) knots -1 -1 -1 -1 -1 -1 -0.98571429 -0.97142857 -0.95714286 -0.94285714 -0.92857143 -0.91428571 -0.9 -0.88571429 -0.87142857 -0.85714286 -0.84285714 -0.82857143 -0.81428571 -0.8 -0.78571429 -0.77142857 -0.75714286 -0.74285714 -0.72857143 -0.71428571 -0.7 -0.68571429 -0.67142857 -0.65714286 -0.64285714 -0.62857143 -0.61428571 -0.6 -0.58571429 -0.57142857 -0.55714286 -0.54285714 -0.52857143 -0.51428571 -0.5 -0.48571429 -0.47142857 -0.45714286 -0.44285714 -0.42857143 -0.41428571 -0.4 -0.38571429 -0.37142857 -0.35714286 -0.34285714 -0.32857143 -0.31428571 -0.3 -0.28571429 -0.27142857 -0.25714286 -0.24285714 -0.22857143 -0.21428571 -0.2 -0.18571429 -0.17142857 -0.15714286 -0.14285714 -0.12857143 -0.11428571 -0.1 -0.08571429 -0.07142857 -0.05714286 -0.04285714 -0.02857143 -0.01428571 0 0 0 0 0 0
  line L7 (60.8996, 57.2425) -> (59.8002, 56.2305)
  arc A15 (58.6839, 56.2712) -> (59.8002, 56.2305) centre (59.2626, 56.8145) ccw
  arc A16 (58.6839, 56.2712) -> (55.0627, 59.8924) centre (-0.5538, 0.6546) ccw
  arc A17 (55.022, 61.0086) -> (55.0627, 59.8924) centre (55.606, 60.4711) ccw
  line L8 (55.022, 61.0086) -> (56.034, 62.108)
  spline S8 degree 5 poles (56.034, 62.108) (56.0575, 62.1335) (56.1038, 62.185) (56.1712, 62.2638) (56.2574, 62.3719) (56.3602, 62.5112) (56.4594, 62.6534) (56.5563, 62.7974) (56.6521, 62.9424) (56.747, 63.0881) (56.841, 63.2344) (56.9339, 63.3816) (57.0253, 63.53) (57.1148, 63.6797) (57.2026, 63.8309) (57.2886, 63.9832) (57.3733, 64.1366) (57.4567, 64.2909) (57.5391, 64.4459) (57.6205, 64.6017) (57.7009, 64.7581) (57.7803, 64.9152) (57.8585, 65.0731) (57.9355, 65.2318) (58.0115, 65.3913) (58.0863, 65.5515) (58.1601, 65.7124) (58.2329, 65.8739) (58.3048, 66.0361) (58.3757, 66.1989) (58.4457, 66.3622) (58.5147, 66.5262) (58.5829, 66.6907) (58.65, 66.8559) (58.7163, 67.0216) (58.7816, 67.1879) (58.8461, 67.3547) (58.9096, 67.522) (58.9723, 67.6899) (59.0342, 67.8583) (59.0952, 68.0271) (59.1553, 68.1965) (59.2146, 68.3663) (59.2731, 68.5367) (59.3307, 68.7075) (59.3876, 68.8787) (59.4436, 69.0505) (59.4988, 69.2226) (59.5532, 69.3952) (59.6068, 69.5683) (59.6596, 69.7417) (59.7116, 69.9156) (59.7628, 70.0899) (59.8133, 70.2647) (59.863, 70.4398) (59.912, 70.6153) (59.9601, 70.7912) (60.0075, 70.9675) (60.0542, 71.1442) (60.1001, 71.3212) (60.1453, 71.4986) (60.1897, 71.6764) (60.2334, 71.8546) (60.2764, 72.0331) (60.3186, 72.212) (60.3601, 72.3912) (60.4009, 72.5707) (60.441, 72.7506) (60.4803, 72.9308) (60.5189, 73.1113) (60.5569, 73.2922) (60.5866, 73.4372) (60.6086, 73.546) (60.6232, 73.6187) (60.6304, 73.655) knots 0 0 0 0 0 0 0.01428571 0.02857143 0.04285714 0.05714286 0.07142857 0.08571429 0.1 0.11428571 0.12857143 0.14285714 0.15714286 0.17142857 0.18571429 0.2 0.21428571 0.22857143 0.24285714 0.25714286 0.27142857 0.28571429 0.3 0.31428571 0.32857143 0.34285714 0.35714286 0.37142857 0.38571429 0.4 0.41428571 0.42857143 0.44285714 0.45714286 0.47142857 0.48571429 0.5 0.51428571 0.52857143 0.54285714 0.55714286 0.57142857 0.58571429 0.6 0.61428571 0.62857143 0.64285714 0.65714286 0.67142857 0.68571429 0.7 0.71428571 0.72857143 0.74285714 0.75714286 0.77142857 0.78571429 0.8 0.81428571 0.82857143 0.84285714 0.85714286 0.87142857 0.88571429 0.9 0.91428571 0.92857143 0.94285714 0.95714286 0.97142857 0.98571429 1 1 1 1 1 1
  arc A18 (60.6304, 73.655) -> (57.0015, 76.549) centre (-0.5538, 0.6546) ccw
  spline S9 degree 5 poles (57.0015, 76.549) (56.9677, 76.5338) (56.9001, 76.5035) (56.7988, 76.4578) (56.6641, 76.3965) (56.4962, 76.3193) (56.3288, 76.2415) (56.1619, 76.163) (55.9954, 76.0839) (55.8295, 76.0042) (55.664, 75.9239) (55.499, 75.8429) (55.3345, 75.7613) (55.1706, 75.6791) (55.0071, 75.5962) (54.8442, 75.5127) (54.6818, 75.4285) (54.5199, 75.3437) (54.3586, 75.2583) (54.1978, 75.1721) (54.0376, 75.0854) (53.878, 74.998) (53.7188, 74.9099) (53.5603, 74.8211) (53.4024, 74.7317) (53.245, 74.6416) (53.0882, 74.5508) (52.932, 74.4594) (52.7765, 74.3673) (52.6215, 74.2745) (52.4672, 74.181) (52.3135, 74.0868) (52.1604, 73.9919) (52.0081, 73.8962) (51.8563, 73.7999) (51.7053, 73.7029) (51.5549, 73.6051) (51.4052, 73.5066) (51.2562, 73.4074) (51.1079, 73.3075) (50.9603, 73.2068) (50.8135, 73.1053) (50.6674, 73.0031) (50.5222, 72.9) (50.3777, 72.7962) (50.234, 72.6917) (50.0911, 72.5863) (49.949, 72.4802) (49.8077, 72.3732) (49.6672, 72.2655) (49.5277, 72.1569) (49.3891, 72.0473) (49.2516, 71.9369) (49.115, 71.8255) (48.9795, 71.7132) (48.8449, 71.6) (48.7112, 71.486) (48.5784, 71.3712) (48.4465, 71.2555) (48.3158, 71.1388) (48.1864, 71.021) (48.0586, 70.9018) (47.9325, 70.7812) (47.8082, 70.6591) (47.6854, 70.5358) (47.5636, 70.4116) (47.4428, 70.2866) (47.3227, 70.161) (47.2038, 70.0344) (47.0872, 69.9061) (46.9744, 69.7749) (46.8882, 69.6668) (46.8263, 69.5835) (46.7864, 69.527) (46.7668, 69.4984) knots -1 -1 -1 -1 -1 -1 -0.98571429 -0.97142857 -0.95714286 -0.94285714 -0.92857143 -0.91428571 -0.9 -0.88571429 -0.87142857 -0.85714286 -0.84285714 -0.82857143 -0.81428571 -0.8 -0.78571429 -0.77142857 -0.75714286 -0.74285714 -0.72857143 -0.71428571 -0.7 -0.68571429 -0.67142857 -0.65714286 -0.64285714 -0.62857143 -0.61428571 -0.6 -0.58571429 -0.57142857 -0.55714286 -0.54285714 -0.52857143 -0.51428571 -0.5 -0.48571429 -0.47142857 -0.45714286 -0.44285714 -0.42857143 -0.41428571 -0.4 -0.38571429 -0.37142857 -0.35714286 -0.34285714 -0.32857143 -0.31428571 -0.3 -0.28571429 -0.27142857 -0.25714286 -0.24285714 -0.22857143 -0.21428571 -0.2 -0.18571429 -0.17142857 -0.15714286 -0.14285714 -0.12857143 -0.11428571 -0.1 -0.08571429 -0.07142857 -0.05714286 -0.04285714 -0.02857143 -0.01428571 0 0 0 0 0 0
  line L9 (46.7668, 69.4984) -> (45.9202, 68.2671)
  arc A19 (44.8229, 68.0584) -> (45.9202, 68.2671) centre (45.2661, 68.7168) ccw
  arc A20 (44.8229, 68.0584) -> (40.4866, 70.783) centre (-0.5538, 0.6546) ccw
  arc A21 (40.1986, 71.8622) -> (40.4866, 70.783) centre (40.8875, 71.4681) ccw
  line L10 (40.1986, 71.8622) -> (40.9406, 73.1593)
  spline S10 degree 5 poles (40.9406, 73.1593) (40.9578, 73.1893) (40.9914, 73.2498) (41.0397, 73.3417) (41.0997, 73.4662) (41.1689, 73.6249) (41.2339, 73.7856) (41.2964, 73.9476) (41.3574, 74.1103) (41.4176, 74.2734) (41.4767, 74.437) (41.5345, 74.6011) (41.5906, 74.7661) (41.6445, 74.9321) (41.6965, 75.0989) (41.7465, 75.2666) (41.7949, 75.435) (41.8419, 75.604) (41.8877, 75.7735) (41.9324, 75.9434) (41.976, 76.1138) (42.0184, 76.2846) (42.0595, 76.456) (42.0993, 76.6278) (42.1379, 76.8002) (42.1752, 76.973) (42.2113, 77.1463) (42.2464, 77.32) (42.2803, 77.4941) (42.3133, 77.6686) (42.3451, 77.8434) (42.376, 78.0187) (42.4058, 78.1942) (42.4345, 78.3702) (42.4622, 78.5465) (42.4889, 78.7231) (42.5146, 78.9001) (42.5394, 79.0774) (42.5631, 79.255) (42.586, 79.4329) (42.6079, 79.6111) (42.6288, 79.7896) (42.6488, 79.9684) (42.6679, 80.1475) (42.6861, 80.3268) (42.7034, 80.5064) (42.7198, 80.6863) (42.7353, 80.8664) (42.7499, 81.0468) (42.7637, 81.2275) (42.7766, 81.4083) (42.7886, 81.5894) (42.7998, 81.7708) (42.8101, 81.9523) (42.8196, 82.1341) (42.8282, 82.3161) (42.8361, 82.4984) (42.8431, 82.6808) (42.8492, 82.8634) (42.8546, 83.0462) (42.8592, 83.2293) (42.8629, 83.4125) (42.8659, 83.5959) (42.868, 83.7795) (42.8694, 83.9633) (42.87, 84.1472) (42.8698, 84.3313) (42.8688, 84.5156) (42.8671, 84.7001) (42.8646, 84.8847) (42.8613, 85.0694) (42.8581, 85.2174) (42.8553, 85.3284) (42.8533, 85.4025) (42.8523, 85.4395) knots 0 0 0 0 0 0 0.01428571 0.02857143 0.04285714 0.05714286 0.07142857 0.08571429 0.1 0.11428571 0.12857143 0.14285714 0.15714286 0.17142857 0.18571429 0.2 0.21428571 0.22857143 0.24285714 0.25714286 0.27142857 0.28571429 0.3 0.31428571 0.32857143 0.34285714 0.35714286 0.37142857 0.38571429 0.4 0.41428571 0.42857143 0.44285714 0.45714286 0.47142857 0.48571429 0.5 0.51428571 0.52857143 0.54285714 0.55714286 0.57142857 0.58571429 0.6 0.61428571 0.62857143 0.64285714 0.65714286 0.67142857 0.68571429 0.7 0.71428571 0.72857143 0.74285714 0.75714286 0.77142857 0.78571429 0.8 0.81428571 0.82857143 0.84285714 0.85714286 0.87142857 0.88571429 0.9 0.91428571 0.92857143 0.94285714 0.95714286 0.97142857 0.98571429 1 1 1 1 1 1
  arc A22 (42.8523, 85.4395) -> (38.6704, 87.4534) centre (-0.5538, 0.6546) ccw
  spline S11 degree 5 poles (38.6704, 87.4534) (38.6408, 87.4311) (38.5816, 87.3865) (38.4931, 87.3194) (38.3754, 87.2297) (38.2289, 87.1171) (38.083, 87.0039) (37.9377, 86.8903) (37.793, 86.7762) (37.649, 86.6615) (37.5055, 86.5464) (37.3627, 86.4307) (37.2205, 86.3146) (37.0789, 86.1979) (36.938, 86.0807) (36.7978, 85.9631) (36.6582, 85.8449) (36.5193, 85.7262) (36.381, 85.607) (36.2434, 85.4872) (36.1065, 85.367) (35.9703, 85.2462) (35.8348, 85.1249) (35.7, 85.0031) (35.5659, 84.8808) (35.4325, 84.758) (35.2998, 84.6346) (35.1679, 84.5107) (35.0368, 84.3863) (34.9063, 84.2613) (34.7767, 84.1358) (34.6478, 84.0098) (34.5197, 83.8832) (34.3924, 83.756) (34.2659, 83.6284) (34.1403, 83.5001) (34.0154, 83.3714) (33.8914, 83.242) (33.7682, 83.1122) (33.6458, 82.9817) (33.5244, 82.8507) (33.4038, 82.7191) (33.2842, 82.587) (33.1655, 82.4542) (33.0477, 82.3208) (32.9309, 82.1869) (32.815, 82.0524) (32.7001, 81.9173) (32.5861, 81.7816) (32.4732, 81.6453) (32.3613, 81.5083) (32.2506, 81.3707) (32.141, 81.2324) (32.0327, 81.0935) (31.9255, 80.9538) (31.8195, 80.8135) (31.7145, 80.6726) (31.6106, 80.5311) (31.5078, 80.389) (31.4063, 80.2462) (31.3064, 80.1025) (31.2083, 79.9579) (31.1123, 79.8122) (31.0182, 79.6655) (30.9259, 79.518) (30.8349, 79.3697) (30.7448, 79.221) (30.6557, 79.0719) (30.568, 78.922) (30.4829, 78.771) (30.402, 78.618) (30.342, 78.4934) (30.3003, 78.3984) (30.274, 78.3344) (30.2612, 78.3022) knots -1 -1 -1 -1 -1 -1 -0.98571429 -0.97142857 -0.95714286 -0.94285714 -0.92857143 -0.91428571 -0.9 -0.88571429 -0.87142857 -0.85714286 -0.84285714 -0.82857143 -0.81428571 -0.8 -0.78571429 -0.77142857 -0.75714286 -0.74285714 -0.72857143 -0.71428571 -0.7 -0.68571429 -0.67142857 -0.65714286 -0.64285714 -0.62857143 -0.61428571 -0.6 -0.58571429 -0.57142857 -0.55714286 -0.54285714 -0.52857143 -0.51428571 -0.5 -0.48571429 -0.47142857 -0.45714286 -0.44285714 -0.42857143 -0.41428571 -0.4 -0.38571429 -0.37142857 -0.35714286 -0.34285714 -0.32857143 -0.31428571 -0.3 -0.28571429 -0.27142857 -0.25714286 -0.24285714 -0.22857143 -0.21428571 -0.2 -0.18571429 -0.17142857 -0.15714286 -0.14285714 -0.12857143 -0.11428571 -0.1 -0.08571429 -0.07142857 -0.05714286 -0.04285714 -0.02857143 -0.01428571 0 0 0 0 0 0
  line L11 (30.2612, 78.3022) -> (29.7098, 76.9134)
  arc A23 (28.6864, 76.4657) -> (29.7098, 76.9134) centre (28.9721, 77.2063) ccw
  arc A24 (28.6864, 76.4657) -> (23.8526, 78.1571) centre (-0.5538, 0.6546) ccw
  arc A25 (23.3316, 79.1452) -> (23.8526, 78.1571) centre (24.091, 78.9142) ccw
  line L12 (23.3316, 79.1452) -> (23.7664, 80.5748)
  spline S12 degree 5 poles (23.7664, 80.5748) (23.7765, 80.6079) (23.7959, 80.6744) (23.8224, 80.7747) (23.8532, 80.9095) (23.8854, 81.0795) (23.913, 81.2507) (23.9379, 81.4225) (23.9612, 81.5947) (23.9836, 81.7671) (24.0048, 81.9398) (24.0246, 82.1127) (24.0425, 82.286) (24.0582, 82.4598) (24.0717, 82.634) (24.0832, 82.8086) (24.0929, 82.9836) (24.1011, 83.1588) (24.1081, 83.3342) (24.1139, 83.5098) (24.1185, 83.6856) (24.1218, 83.8616) (24.1237, 84.0378) (24.1243, 84.2142) (24.1235, 84.3909) (24.1214, 84.5677) (24.1181, 84.7447) (24.1136, 84.9218) (24.108, 85.0991) (24.1013, 85.2765) (24.0934, 85.4541) (24.0845, 85.6318) (24.0745, 85.8096) (24.0634, 85.9875) (24.0512, 86.1655) (24.0379, 86.3437) (24.0236, 86.522) (24.0082, 86.7003) (23.9919, 86.8787) (23.9746, 87.0573) (23.9562, 87.2359) (23.9369, 87.4146) (23.9167, 87.5933) (23.8955, 87.7722) (23.8733, 87.9511) (23.8502, 88.13) (23.8261, 88.309) (23.8011, 88.4881) (23.7753, 88.6672) (23.7485, 88.8464) (23.7208, 89.0256) (23.6922, 89.2048) (23.6628, 89.3841) (23.6324, 89.5634) (23.6012, 89.7428) (23.5692, 89.9221) (23.5362, 90.1015) (23.5025, 90.2809) (23.4679, 90.4604) (23.4324, 90.6398) (23.3961, 90.8193) (23.359, 90.9987) (23.3211, 91.1782) (23.2823, 91.3576) (23.2428, 91.5371) (23.2024, 91.7166) (23.1613, 91.896) (23.1193, 92.0755) (23.0766, 92.2549) (23.033, 92.4344) (22.9887, 92.6138) (22.9527, 92.7573) (22.9253, 92.8649) (22.9068, 92.9367) (22.8976, 92.9725) knots 0 0 0 0 0 0 0.01428571 0.02857143 0.04285714 0.05714286 0.07142857 0.08571429 0.1 0.11428571 0.12857143 0.14285714 0.15714286 0.17142857 0.18571429 0.2 0.21428571 0.22857143 0.24285714 0.25714286 0.27142857 0.28571429 0.3 0.31428571 0.32857143 0.34285714 0.35714286 0.37142857 0.38571429 0.4 0.41428571 0.42857143 0.44285714 0.45714286 0.47142857 0.48571429 0.5 0.51428571 0.52857143 0.54285714 0.55714286 0.57142857 0.58571429 0.6 0.61428571 0.62857143 0.64285714 0.65714286 0.67142857 0.68571429 0.7 0.71428571 0.72857143 0.74285714 0.75714286 0.77142857 0.78571429 0.8 0.81428571 0.82857143 0.84285714 0.85714286 0.87142857 0.88571429 0.9 0.91428571 0.92857143 0.94285714 0.95714286 0.97142857 0.98571429 1 1 1 1 1 1
  arc A26 (22.8976, 92.9725) -> (18.3724, 94.0054) centre (-0.5538, 0.6546) ccw
  spline S13 degree 5 poles (18.3724, 94.0054) (18.3485, 93.9771) (18.3008, 93.9204) (18.2294, 93.8353) (18.1346, 93.7217) (18.0168, 93.5793) (17.8998, 93.4365) (17.7834, 93.2934) (17.6677, 93.1499) (17.5528, 93.0061) (17.4386, 92.8619) (17.3251, 92.7174) (17.2123, 92.5725) (17.1002, 92.4272) (16.9889, 92.2817) (16.8784, 92.1357) (16.7686, 91.9894) (16.6596, 91.8428) (16.5513, 91.6958) (16.4438, 91.5485) (16.3371, 91.4008) (16.2312, 91.2527) (16.126, 91.1043) (16.0217, 90.9556) (15.9182, 90.8065) (15.8155, 90.657) (15.7136, 90.5072) (15.6126, 90.3571) (15.5124, 90.2066) (15.4131, 90.0557) (15.3146, 89.9045) (15.217, 89.753) (15.1203, 89.6011) (15.0244, 89.4488) (14.9295, 89.2962) (14.8355, 89.1432) (14.7425, 88.9899) (14.6503, 88.8362) (14.5591, 88.6822) (14.4689, 88.5278) (14.3796, 88.373) (14.2914, 88.2179) (14.2041, 88.0624) (14.118, 87.9066) (14.0328, 87.7503) (13.9487, 87.5938) (13.8657, 87.4368) (13.7837, 87.2796) (13.7028, 87.1219) (13.623, 86.9639) (13.5444, 86.8055) (13.4671, 86.6467) (13.3911, 86.4875) (13.3164, 86.3279) (13.243, 86.1679) (13.1708, 86.0075) (13.0998, 85.8468) (13.03, 85.6857) (12.9614, 85.5243) (12.8942, 85.3624) (12.8288, 85.2001) (12.7654, 85.0373) (12.7041, 84.8739) (12.645, 84.71) (12.5879, 84.5456) (12.5321, 84.3808) (12.4774, 84.2158) (12.4237, 84.0505) (12.3716, 83.8849) (12.3222, 83.7188) (12.2774, 83.5516) (12.2467, 83.4168) (12.2271, 83.3149) (12.2157, 83.2466) (12.2104, 83.2124) knots -1 -1 -1 -1 -1 -1 -0.98571429 -0.97142857 -0.95714286 -0.94285714 -0.92857143 -0.91428571 -0.9 -0.88571429 -0.87142857 -0.85714286 -0.84285714 -0.82857143 -0.81428571 -0.8 -0.78571429 -0.77142857 -0.75714286 -0.74285714 -0.72857143 -0.71428571 -0.7 -0.68571429 -0.67142857 -0.65714286 -0.64285714 -0.62857143 -0.61428571 -0.6 -0.58571429 -0.57142857 -0.55714286 -0.54285714 -0.52857143 -0.51428571 -0.5 -0.48571429 -0.47142857 -0.45714286 -0.44285714 -0.42857143 -0.41428571 -0.4 -0.38571429 -0.37142857 -0.35714286 -0.34285714 -0.32857143 -0.31428571 -0.3 -0.28571429 -0.27142857 -0.25714286 -0.24285714 -0.22857143 -0.21428571 -0.2 -0.18571429 -0.17142857 -0.15714286 -0.14285714 -0.12857143 -0.11428571 -0.1 -0.08571429 -0.07142857 -0.05714286 -0.04285714 -0.02857143 -0.01428571 0 0 0 0 0 0
  line L13 (12.2104, 83.2124) -> (11.9819, 81.7357)
  arc A27 (11.0838, 81.0715) -> (11.9819, 81.7357) centre (11.1974, 81.8571) ccw
  arc A28 (11.0838, 81.0715) -> (5.9948, 81.6449) centre (-0.5538, 0.6546) ccw
  arc A29 (5.267, 82.4923) -> (5.9948, 81.6449) centre (6.0588, 82.4361) ccw
  line L14 (5.267, 82.4923) -> (5.3728, 83.9828)
  spline S14 degree 5 poles (5.3728, 83.9828) (5.3752, 84.0174) (5.3793, 84.0864) (5.3829, 84.1901) (5.3829, 84.3284) (5.3764, 84.5014) (5.3653, 84.6744) (5.3513, 84.8474) (5.3357, 85.0205) (5.3191, 85.1935) (5.3014, 85.3666) (5.2823, 85.5396) (5.2612, 85.7126) (5.2378, 85.8855) (5.2122, 86.0583) (5.1845, 86.2311) (5.155, 86.4038) (5.1241, 86.5765) (5.0918, 86.7491) (5.0584, 86.9216) (5.0237, 87.094) (4.9878, 87.2663) (4.9505, 87.4385) (4.9118, 87.6106) (4.8717, 87.7827) (4.8304, 87.9546) (4.7877, 88.1264) (4.7439, 88.2981) (4.699, 88.4697) (4.653, 88.6412) (4.6058, 88.8125) (4.5576, 88.9838) (4.5082, 89.1549) (4.4578, 89.3259) (4.4063, 89.4967) (4.3537, 89.6675) (4.3001, 89.8381) (4.2454, 90.0085) (4.1898, 90.1789) (4.1332, 90.3491) (4.0756, 90.5191) (4.017, 90.689) (3.9575, 90.8588) (3.897, 91.0284) (3.8356, 91.1979) (3.7732, 91.3672) (3.7099, 91.5364) (3.6457, 91.7054) (3.5806, 91.8743) (3.5147, 92.043) (3.4478, 92.2116) (3.3801, 92.38) (3.3114, 92.5482) (3.242, 92.7162) (3.1716, 92.8842) (3.1005, 93.0519) (3.0285, 93.2195) (2.9556, 93.3869) (2.8819, 93.5541) (2.8074, 93.7211) (2.7321, 93.888) (2.656, 94.0547) (2.5791, 94.2212) (2.5014, 94.3876) (2.4229, 94.5538) (2.3436, 94.7197) (2.2636, 94.8855) (2.1827, 95.0512) (2.1011, 95.2166) (2.0188, 95.3818) (1.9356, 95.5469) (1.8685, 95.6788) (1.8179, 95.7776) (1.7839, 95.8434) (1.7669, 95.8764) knots 0 0 0 0 0 0 0.01428571 0.02857143 0.04285714 0.05714286 0.07142857 0.08571429 0.1 0.11428571 0.12857143 0.14285714 0.15714286 0.17142857 0.18571429 0.2 0.21428571 0.22857143 0.24285714 0.25714286 0.27142857 0.28571429 0.3 0.31428571 0.32857143 0.34285714 0.35714286 0.37142857 0.38571429 0.4 0.41428571 0.42857143 0.44285714 0.45714286 0.47142857 0.48571429 0.5 0.51428571 0.52857143 0.54285714 0.55714286 0.57142857 0.58571429 0.6 0.61428571 0.62857143 0.64285714 0.65714286 0.67142857 0.68571429 0.7 0.71428571 0.72857143 0.74285714 0.75714286 0.77142857 0.78571429 0.8 0.81428571 0.82857143 0.84285714 0.85714286 0.87142857 0.88571429 0.9 0.91428571 0.92857143 0.94285714 0.95714286 0.97142857 0.98571429 1 1 1 1 1 1